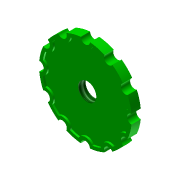
# Autodesk Inventor part: Tripod_Wheel
Saved by Autodesk Inventor 2012 (Build 160160000, 160)
## iProperties
Created: 2012-06-04
Part Number: Tripod_Wheel
Material: Polypropylene
Document SubType Name: Modeling
Designer: Lee
Mass: 0.871985 g
Surface Area: 12.3236 cm^2
Volume: 0.96995 cm^3
Density: 0.899 g/cm^3
Author: Lee
Autodesk Inventor part; units mm, degrees
ref_plane "YZ Plane" through (0, 0, 0) normal (1, 0, 0) x (0, 1, 0)
ref_plane "XZ Plane" through (0, 0, 0) normal (0, 1, 0) x (-1, 0, 0)
ref_plane "XY Plane" through (0, 0, 0) normal (0, 0, 1) x (1, 0, 0)
sketch "Sketch1" plane through (0, 0, 0) normal (0, 0, 1) x (1, 0, 0)
  circle A0 centre (0, 0) radius 12.7
  dimension "d9" = 25.4
  constraints: 1 centre point, 1 coincident
  measures "d9" diameter of A0
extrude "Extrusion1" add sketch "Sketch1" along normal blind 2.54
sketch "Sketch2" plane through (0, 0, 2.54) normal (0, 0, 1) x (1, 0, 0)
  circle A0 centre (0, 12.7) radius 1.27
  dimension "d12" = 2.54
  constraints: 1 centre point
  measures "d12" diameter of A0
extrude "Extrusion2" cut sketch "Sketch2" against normal through all
pattern_circular "Circular Pattern1" count 12 over 360 about axis through (0, 0, 0) along (0, 0, 1) of "Extrusion2"
sketch "Sketch3" plane through (0, 0, 2.54) normal (0, 0, 1) x (1, 0, 0)
  arc A0 (5.2198, 11.5777) -> (7.4167, 10.3093) centre (6.35, 10.9985) ccw projected
  arc A1 (5.2198, 11.5777) -> (1.2684, 12.6365) centre (0, 0) ccw projected
  arc A2 (-1.2684, 12.6365) -> (1.2684, 12.6365) centre (0, 12.7) ccw projected
  arc A3 (-1.2684, 12.6365) -> (-5.2198, 11.5777) centre (0, 0) ccw projected
  arc A4 (-7.4167, 10.3093) -> (-5.2198, 11.5777) centre (-6.35, 10.9985) ccw projected
  arc A5 (-7.4167, 10.3093) -> (-10.3093, 7.4167) centre (0, 0) ccw projected
  arc A6 (-11.5777, 5.2198) -> (-10.3093, 7.4167) centre (-10.9985, 6.35) ccw projected
  arc A7 (-11.5777, 5.2198) -> (-12.6365, 1.2684) centre (0, 0) ccw projected
  arc A8 (-12.6365, -1.2684) -> (-12.6365, 1.2684) centre (-12.7, 0) ccw projected
  arc A9 (-12.6365, -1.2684) -> (-11.5777, -5.2198) centre (0, 0) ccw projected
  arc A10 (-10.3093, -7.4167) -> (-11.5777, -5.2198) centre (-10.9985, -6.35) ccw projected
  arc A11 (-10.3093, -7.4167) -> (-7.4167, -10.3093) centre (0, 0) ccw projected
  arc A12 (-5.2198, -11.5777) -> (-7.4167, -10.3093) centre (-6.35, -10.9985) ccw projected
  arc A13 (-5.2198, -11.5777) -> (-1.2684, -12.6365) centre (0, 0) ccw projected
  arc A14 (1.2684, -12.6365) -> (-1.2684, -12.6365) centre (0, -12.7) ccw projected
  arc A15 (1.2684, -12.6365) -> (5.2198, -11.5777) centre (0, 0) ccw projected
  arc A16 (7.4167, -10.3093) -> (5.2198, -11.5777) centre (6.35, -10.9985) ccw projected
  arc A17 (7.4167, -10.3093) -> (10.3093, -7.4167) centre (0, 0) ccw projected
  arc A18 (11.5777, -5.2198) -> (10.3093, -7.4167) centre (10.9985, -6.35) ccw projected
  arc A19 (11.5777, -5.2198) -> (12.6365, -1.2684) centre (0, 0) ccw projected
  arc A20 (12.6365, 1.2684) -> (12.6365, -1.2684) centre (12.7, 0) ccw projected
  arc A21 (12.6365, 1.2684) -> (11.5777, 5.2198) centre (0, 0) ccw projected
  arc A22 (10.3093, 7.4167) -> (11.5777, 5.2198) centre (10.9985, 6.35) ccw projected
  arc A23 (10.3093, 7.4167) -> (7.4167, 10.3093) centre (0, 0) ccw projected
  arc A24 (-1.8912, 11.6586) -> (-4.1914, 11.0423) centre (0, 0) ccw
  arc A25 (-1.8912, 11.6586) -> (1.8912, 11.6586) centre (0, 12.7) ccw
  arc A26 (4.1914, 11.0423) -> (1.8912, 11.6586) centre (0, 0) ccw
  arc A27 (4.1914, 11.0423) -> (7.4672, 9.151) centre (6.35, 10.9985) ccw
  arc A28 (9.151, 7.4672) -> (7.4672, 9.151) centre (0, 0) ccw
  arc A29 (9.151, 7.4672) -> (11.0423, 4.1914) centre (10.9985, 6.35) ccw
  arc A30 (11.6586, 1.8912) -> (11.0423, 4.1914) centre (0, 0) ccw
  arc A31 (11.6586, 1.8912) -> (11.6586, -1.8912) centre (12.7, 0) ccw
  arc A32 (11.0423, -4.1914) -> (11.6586, -1.8912) centre (0, 0) ccw
  arc A33 (11.0423, -4.1914) -> (9.151, -7.4672) centre (10.9985, -6.35) ccw
  arc A34 (7.4672, -9.151) -> (9.151, -7.4672) centre (0, 0) ccw
  arc A35 (7.4672, -9.151) -> (4.1914, -11.0423) centre (6.35, -10.9985) ccw
  arc A36 (1.8912, -11.6586) -> (4.1914, -11.0423) centre (0, 0) ccw
  arc A37 (1.8912, -11.6586) -> (-1.8912, -11.6586) centre (0, -12.7) ccw
  arc A38 (-4.1914, -11.0423) -> (-1.8912, -11.6586) centre (0, 0) ccw
  arc A39 (-4.1914, -11.0423) -> (-7.4672, -9.151) centre (-6.35, -10.9985) ccw
  arc A40 (-9.151, -7.4672) -> (-7.4672, -9.151) centre (0, 0) ccw
  arc A41 (-9.151, -7.4672) -> (-11.0423, -4.1914) centre (-10.9985, -6.35) ccw
  arc A42 (-11.6586, -1.8912) -> (-11.0423, -4.1914) centre (0, 0) ccw
  arc A43 (-11.6586, -1.8912) -> (-11.6586, 1.8912) centre (-12.7, 0) ccw
  arc A44 (-11.0423, 4.1914) -> (-11.6586, 1.8912) centre (0, 0) ccw
  arc A45 (-11.0423, 4.1914) -> (-9.151, 7.4672) centre (-10.9985, 6.35) ccw
  arc A46 (-7.4672, 9.151) -> (-9.151, 7.4672) centre (0, 0) ccw
  arc A47 (-7.4672, 9.151) -> (-4.1914, 11.0423) centre (-6.35, 10.9985) ccw
  dimension "d18" = 0.889
  constraints: 48 point on circle, 24 centre point, 23 other
  measures "d18" radial gap between concentric circles of A25 A2
extrude "Extrusion3" cut sketch "Sketch3" against normal blind 0.508 contours A25 A26 A27 A28 A29 A30 A31 A32 A33 A34 A35 A36 A37 A38 A39 A40 A41 A42 A43 A44 A45 A46 A47 A24
hole "Hole1" at (0, 0, 0) direction (0, 0, 1) diameter 4.9784 end through all thread size "1/4-20 UNC" class "2B" standard "ANSI Unified Screw Threads"
body "Solid1"
